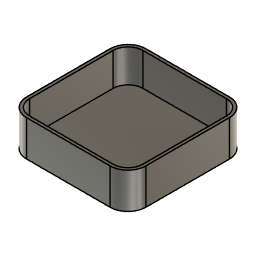
收纳盒 v2 (Autodesk Fusion 360 design; units mm, degrees)
Autodesk Fusion 360 part; units mm, degrees
sketch "草图1" plane through (0, 0, 0) normal (0, 0, 1) x (1, 0, 0)
  line L0 (0, 0) -> (200, 0)
  line L1 (200, 0) -> (200, 200)
  line L2 (200, 200) -> (0, 200)
  line L3 (0, 200) -> (0, 0)
  dimension "d1" = 200
  dimension "d2" = 200
  constraint horizontal L0
  constraint vertical L1
  constraint horizontal L2
  constraint vertical L3
  constraint coincident L0.start L3.end
  measures "d1" distance of L0 L2
  measures "d2" distance of L1 L3
extrude "拉伸1" add sketch "草图1" along normal blind 50
fillet "圆角1" radius 30 4 edges at (0, 0, 25) (200, 0, 25) (200, 200, 25) (0, 200, 25)
shell "抽壳1" thickness 5 removed faces 1 at (123.3333, 86.6667, 50)
extrude "拉伸2" add 1 faces at (76.6667, 1.6667, 50) along direction (0, 0, 1) blind 10
